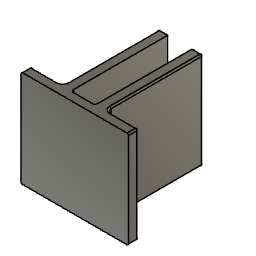
Support vertical ordinateur (Autodesk Fusion 360 design; units mm, degrees)
Autodesk Fusion 360 part; units mm, degrees
sketch "Esquisse1" plane through (0, 0, 0) normal (0, 0, 1) x (1, 0, 0)
  line L0 (0, 10) -> (-12.5, 10)
  line L1 (-12.5, 10) -> (-12.5, 110)
  line L2 (-12.5, 110) -> (-22.5, 110)
  line L3 (-22.5, 110) -> (-22.5, 10)
  line L4 (-22.5, 10) -> (-55.5, 10)
  line L5 (-55.5, 10) -> (-55.5, 0)
  line L6 (-55.5, 0) -> (0, 0)
  line L7 (0, 1.75) -> (0, 22.5)
  line L8 (1.75, 0) -> (22.5, 0)
  line L9 (0, 10) -> (12.5, 10)
  line L10 (12.5, 10) -> (12.5, 110)
  line L11 (12.5, 110) -> (22.5, 110)
  line L12 (22.5, 110) -> (22.5, 10)
  line L13 (22.5, 10) -> (55.5, 10)
  line L14 (55.5, 10) -> (55.5, 0)
  line L15 (55.5, 0) -> (0, 0)
  dimension "d13" = 12.5
  dimension "d15" = 10
  dimension "d16" = 10
  dimension "d17" = 100
  dimension "d19" = 10
  dimension "d20" = 55.5
  constraint horizontal L0
  constraint perpendicular L0 L1
  constraint perpendicular L1 L2
  constraint perpendicular L2 L3
  constraint perpendicular L3 L4
  constraint perpendicular L4 L5
  constraint perpendicular L3 L6
  constraint coincident L6.end L7
  constraint coincident L0.start L7
  constraint coincident L6.end L8
  constraint symmetric L0.start L7 L9.start
  constraint symmetric L0.end L7 L9.end
  constraint symmetric L1.end L7 L10.end
  constraint symmetric L2.end L7 L11.end
  constraint symmetric L3.end L7 L12.end
  constraint symmetric L4.end L7 L13.end
  constraint symmetric L5.end L7 L14.end
  constraint symmetric L6.end L7 L15.end
  measures "d13" distance of L1 L7
  measures "d15" distance of L1 L3
  measures "d16" distance of L4 L8
  measures "d17" distance of L2 L4
  measures "d19" distance of L0 L8
  measures "d20" distance of L5 L7
extrude "Extrusion1" add sketch "Esquisse1" along normal mid plane 100
fillet "Congé5" radius 1.5 1 edges at (55.5, 10, 0)
fillet "Congé5" radius 1.5 1 edges at (-55.5, 10, 0)
fillet "Congé5" radius 1.5 1 edges at (12.5, 10, 0)
fillet "Congé5" radius 1.5 1 edges at (-12.5, 10, 0)
fillet "Congé5" radius 1.5 1 edges at (0, 10, -50)
fillet "Congé5" radius 1.5 1 edges at (0, 10, 50)
fillet "Congé6" radius 5 1 edges at (22.5, 10, 0)
fillet "Congé6" radius 5 1 edges at (-22.5, 10, 0)
fillet "Congé7" radius 1.5 5 edges at (-22.5, 62.5, 50) (-23.9645, 11.4645, 50) (-40.75, 10, 50) (-55.0607, 9.5607, 50) (-55.5, 4.25, 50)
fillet "Congé7" radius 1.5 5 edges at (22.5, 62.5, 50) (23.9645, 11.4645, 50) (40.75, 10, 50) (55.0607, 9.5607, 50) (55.5, 4.25, 50)
fillet "Congé7" radius 1.5 5 edges at (-55.5, 4.25, -50) (-55.0607, 9.5607, -50) (-40.75, 10, -50) (-23.9645, 11.4645, -50) (-22.5, 62.5, -50)
fillet "Congé7" radius 1.5 5 edges at (22.5, 62.5, -50) (23.9645, 11.4645, -50) (40.75, 10, -50) (55.0607, 9.5607, -50) (55.5, 4.25, -50)
fillet "Congé7" radius 1.5 1 edges at (17.5, 110, 50)
fillet "Congé7" radius 1.5 1 edges at (-17.5, 110, 50)
fillet "Congé7" radius 1.5 1 edges at (-17.5, 110, -50)
fillet "Congé7" radius 1.5 1 edges at (17.5, 110, -50)
fillet "Congé7" radius 1.5 4 edges at (22.5, 110, 0) (12.5, 110, 0) (-12.5, 110, 0) (-22.5, 110, 0)
